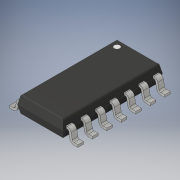
# Autodesk Inventor part: Semiconductor_SOIC-14
Saved by Autodesk Inventor 2017 (Build 210142000, 142)
## iProperties
Created: 2016-07-22
Part Number: Semiconductor_SOIC-14
Material: ABS Plastic
Document SubType Name: Modeling
Designer: Bradley
Density: 1.06 g/cm^3
Appearance: Smooth - Black
Author: Bradley
Autodesk Inventor part; units mm, degrees
ref_plane "YZ Plane" through (0, 0, 0) normal (1, 0, 0) x (0, 1, 0)
ref_plane "XZ Plane" through (0, 0, 0) normal (0, 1, 0) x (-1, 0, 0)
ref_plane "XY Plane" through (0, 0, 0) normal (0, 0, 1) x (1, 0, 0)
sketch "Sketch1" plane through (0, 0, 0) normal (0, 1, 0) x (-1, 0, 0)
  line L0 (-2, 4.375) -> (2, 4.375)
  line L1 (2, 4.375) -> (2, -4.375)
  line L2 (2, -4.375) -> (-2, -4.375)
  line L3 (-2, -4.375) -> (-2, 4.375)
  line L4 (-2, 4.375) -> (2, -4.375) construction
  line L5 (2, 4.375) -> (-2, -4.375) construction
  point P0 (0, 0)
  dimension "d0" = 4
  dimension "d1" = 8.75
  constraints: 12 end point, 2 midpoint, 2 parallel, 1 horizontal, 1 perpendicular
  measures "d0" distance of L1.end L2.end
  measures "d1" distance of L0.end L1.end
extrude "Extrusion1" add sketch "Sketch1" along normal blind 0.75 draft -12
sketch "Sketch2" plane through (0, 0, 0) normal (0, -1, 0) x (1, 0, 0)
  line L0 (2, 4.375) -> (-2, 4.375) projected
  line L1 (2, 4.375) -> (-2, 4.375) projected
  line L2 (-2, 4.375) -> (-2, -4.375) projected
  line L3 (-2, -4.375) -> (2, -4.375) projected
  line L4 (2, -4.375) -> (2, 4.375) projected
  point P0 (0, 0)
extrude "Extrusion2" add sketch "Sketch2" along normal blind 0.75 draft -12
fillet "Fillet1" radius 0.1 8 edges at (-1.8406, 0.75, 0) (0, 0.75, 4.2156) (0, 0.75, -4.2156) (1.8406, 0.75, 0) (1.8406, -0.75, 0) (0, -0.75, 4.2156) (-1.8406, -0.75, 0) (0, -0.75, -4.2156)
sketch "Sketch3" plane through (0, 0, 0) normal (0, 1, 0) x (-1, 0, 0)
  line L0 (2, 4.375) -> (2, -4.375) projected
  line L1 (-2, 4.375) -> (2, 4.375) projected
  line L2 (2, 4.06) -> (2.05, 4.06)
  line L3 (2.05, 4.06) -> (2.05, 3.56)
  line L4 (2.05, 3.56) -> (2, 3.56)
  line L5 (2, 3.56) -> (2, 4.06)
  line L6 (-2, -4.375) -> (-2, 4.375) projected
  line L7 (-2, 4.06) -> (-2.05, 4.06)
  line L8 (-2.05, 4.06) -> (-2.05, 3.56)
  line L9 (-2.05, 3.56) -> (-2, 3.56)
  line L10 (-2, 3.56) -> (-2, 4.06)
  line L11 (-2, 3.56) -> (2, 3.56)
  line L12 (2, 3.56) -> (2, 4.06)
  line L13 (2, 4.06) -> (-2, 4.06)
  line L14 (-2, 4.06) -> (-2, 3.56)
  point P0 (0, 0)
  point P1 (2, 3.81)
  dimension "d7" = 0.5
  dimension "d8" = 3.81
  dimension "d9" = 0.05
  constraints: 24 end point, 6 parallel, 4 point on line, 3 horizontal, 3 perpendicular, 1 collinear, 1 midpoint
  measures "d7" distance of L2.end L3.end
  measures "d8" vertical distance of point (2, 3.81) point (0, 0)
  measures "d9" distance of L3.end L4.end
extrude "Extrusion3" add sketch "Sketch3" along normal blind 0.2 contours L2 L3 L4 L0 | L0 L11 L6 L13 | L6 L9 L8 L7
sketch "Sketch4" plane through (-2.05, 0, 4.06) normal (0, 0, 1) x (1, 0, 0)
  line L0 (0.0925, 0.2) -> (0.05, 0) projected
  line L1 (0, 0.2) -> (0.0925, 0.2) projected
  line L2 (0, 0) -> (0, 0.2) projected
  line L3 (0, 0) -> (0.05, 0) projected
  line L4 (4.05, 0) -> (4.0075, 0.2) projected
  line L5 (4.05, 0) -> (4.1, 0) projected
  line L6 (4.1, 0) -> (4.1, 0.2) projected
  line L7 (4.0075, 0.2) -> (4.1, 0.2) projected
  line L8 (0, 0) -> (0.05, 0) projected
  arc A0 (0, 0) -> (-0.1472, -0.121) centre (0, -0.15) ccw
  arc A1 (-0.5934, -0.925) -> (-0.25, -0.6427) centre (-0.5934, -0.575) ccw
  line L9 (0, 0.2) -> (0.0925, 0.2) projected
  arc A2 (0, 0.2) -> (-0.3434, -0.0823) centre (0, -0.15) ccw
  arc A3 (-0.5934, -0.725) -> (-0.4462, -0.604) centre (-0.5934, -0.575) ccw
  line L10 (-0.5934, -0.925) -> (-0.95, -0.925)
  line L11 (-0.95, -0.925) -> (-0.95, -0.725)
  line L12 (-0.95, -0.725) -> (-0.5934, -0.725)
  line L13 (-0.3434, -0.0823) -> (-0.4462, -0.604)
  line L14 (-0.1472, -0.121) -> (-0.25, -0.6427)
  line L15 (3.8096, -0.75) -> (0.2904, -0.75) projected
  line L16 (0, 0.2) -> (0, 0)
  line L17 (0.2904, 0.75) -> (3.8096, 0.75) projected
  line L18 (2.05, 0.75) -> (2.05, -0.75)
  line L19 (4.1, 0) -> (4.1, 0.2)
  arc A4 (4.2472, -0.121) -> (4.1, 0) centre (4.1, -0.15) ccw
  arc A5 (4.35, -0.6427) -> (4.6934, -0.925) centre (4.6934, -0.575) ccw
  arc A6 (4.4434, -0.0823) -> (4.1, 0.2) centre (4.1, -0.15) ccw
  arc A7 (4.5462, -0.604) -> (4.6934, -0.725) centre (4.6934, -0.575) ccw
  line L20 (4.6934, -0.925) -> (5.05, -0.925)
  line L21 (5.05, -0.925) -> (5.05, -0.725)
  line L22 (5.05, -0.725) -> (4.6934, -0.725)
  line L23 (4.4434, -0.0823) -> (4.5462, -0.604)
  line L24 (4.2472, -0.121) -> (4.35, -0.6427)
  point P0 (2.05, 0)
  dimension "d12" = 0.15
  dimension "d13" = 0.15
  dimension "d16" = 0.7
  dimension "d17" = 0.175
  dimension "d25" = 6
  constraints: 26 end point, 16 point on circle, 12 symmetric about line, 8 centre point, 6 tangent, 4 coincident, 2 equal length, 2 midpoint, 2 perpendicular, 1 horizontal, 1 parallel, 4 other
  measures "d12" radius of A0
  measures "d13" radius of A3
  measures "d16" distance from line of L11 L14.end
  measures "d17" distance between parallel lines of L10 L15
  measures "d25" distance between parallel lines of L21 L11
extrude "Extrusion4" add sketch "Sketch4" against normal up to surface (0.5 mm away) contours L2 A0 L14 A1 L10 L11 L12 A3 L13 A2 | L6 A6 L23 A7 L22 L21 L20 A5 L24 A4
pattern_linear "Rectangular Pattern1" count 7 spacing 1.27 along (0, 0, -1) of "Extrusion4", "Extrusion3"
sketch "Sketch5" plane through (0, 0.75, 0) normal (0, 1, 0) x (1, 0, 0)
  line L0 (1.7596, -4.1346) -> (-1.7596, -4.1346) projected
  line L1 (1.7596, 4.1346) -> (1.7596, -4.1346) projected
  line L2 (-1.7596, 4.1346) -> (1.7596, 4.1346) projected
  line L3 (-1.7596, -4.1346) -> (-1.7596, 4.1346) projected
  circle A0 centre (-1.2596, 3.6346) radius 0.25
  circle A1 centre (-1.2596, 3.6346) radius 0.5 construction
  line L4 (-1.7596, -4.1346) -> (-1.7596, 4.1346) projected
  line L5 (-1.7596, -4.1346) -> (1.7596, -4.1346) construction
  line L6 (-1.7596, 4.1346) -> (1.7596, 4.1346) construction
  point P0 (0, 0)
  dimension "d26" = 1
  dimension "d27" = 0.5
  constraints: 2 centre point, 2 tangent, 1 coincident
  measures "d26" diameter of A1
  measures "d27" diameter of A0
extrude "Extrusion5" add sketch "Sketch5" along normal blind 0.01 contours A0
equation "\"d13\" = d12"
body "Solid1"
